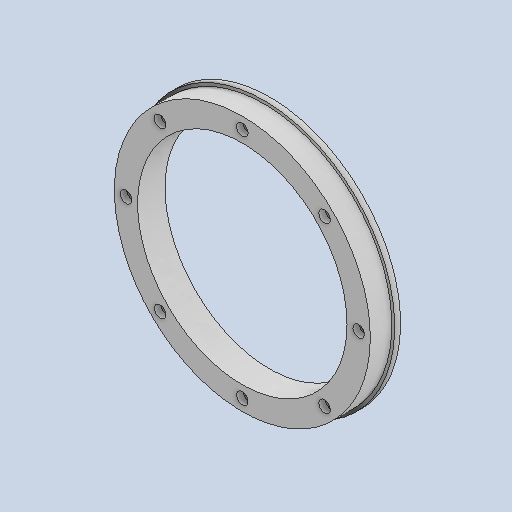
# Autodesk Inventor part: ДМФ 016 Барабан Опорное кольцо КОРМА
Saved by Autodesk Inventor 2024.2 (Build 282272000, 272)
## iProperties
Created: 2024-04-28
Part Number: ДМФ 016 Барабан Опорное кольцо КОРМА
Material: Generic
Document SubType Name: Modeling
Designer: admin
Density: 1 g/cm^3
Appearance: Default
Author: pokla
Autodesk Inventor part; units mm, degrees
ref_plane "YZ Plane" through (0, 0, 0) normal (1, 0, 0) x (0, 1, 0)
ref_plane "XZ Plane" through (0, 0, 0) normal (0, 1, 0) x (-1, 0, 0)
ref_plane "XY Plane" through (0, 0, 0) normal (0, 0, 1) x (1, 0, 0)
sketch "Sketch1" plane through (0, 0, 0) normal (0, 0, 1) x (1, 0, 0)
  circle A0 centre (0, 0) radius 180
  circle A1 centre (0, 0) radius 220
  dimension "d0" = 40
  dimension "d1" = 360
  constraints: 2 centre point, 1 coincident
  measures "d0" radial gap between concentric circles of A0 A1
  measures "d1" diameter of A0
extrude "Extrusion1" add sketch "Sketch1" along normal blind 47
sketch "Sketch2" plane through (0, 0, 47) normal (0, 0, 1) x (1, 0, 0)
  circle A0 centre (0, 0) radius 220 construction
  circle A1 centre (0, 0) radius 180 construction
  line L0 (0, 220) -> (0, 180) construction
  circle A2 centre (0, 200) radius 6.25
  dimension "d4" = 12.5
  constraints: 3 vertical alignment, 2 end point, 1 centre point, 1 coincident, 1 midpoint, 1 vertical, 2 other
  measures "d4" diameter of A2
extrude "Extrusion2" cut sketch "Sketch2" against normal through all
sketch "Sketch3" plane through (0, 0, 47) normal (0, 0, 1) x (1, 0, 0)
  circle A0 centre (0, 200) radius 6.25 projected
  circle A1 centre (0, 200) radius 10
  point P0 (0, 0)
  dimension "d10" = 20
  constraints: 1 centre point
  measures "d10" diameter of A1
extrude "Extrusion3" cut sketch "Sketch3" against normal blind 11
pattern_circular "Circular Pattern1" count 8 over 360 about axis through (0, 0, 0) along (0, 0, 1) of "Extrusion2", "Extrusion3"
sketch "Sketch4" plane through (0, 0, 0) normal (0, 0, -1) x (-1, 0, 0)
  circle A0 centre (0, 0) radius 220 projected
  circle A1 centre (0, 0) radius 225
  dimension "d13" = 5
  constraints: 1 centre point
  measures "d13" radial gap between concentric circles of A0 A1
extrude "Extrusion4" add sketch "Sketch4" against normal blind 10
equation "\"d1\" = Вал_ось_диаметр_КОРМА"
equation "\"d2\" = Барабан_толщина_посад_кольца"
equation "\"Вал_ось_диаметр_КОРМА\" = 360"
equation "\"Барабан_толщина_посад_кольца\" = 47"
body "Solid1"
